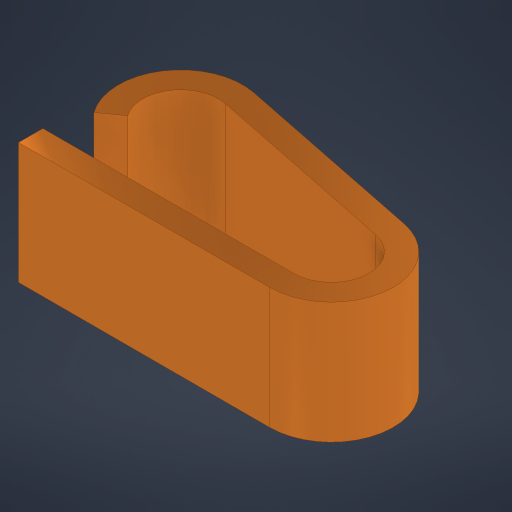
# Autodesk Inventor part: spring contact
Saved by Autodesk Inventor 2024.3 (Build 283343010, 343A)
## iProperties
Created: 2025-05-07
Part Number: spring contact
Material: Gold
Document SubType Name: Modeling
Designer: David
Density: 19.3 g/cm^3
Appearance: Metall - 1600F (heiß)
Author: David
Autodesk Inventor part; units mm, degrees
ref_plane "YZ Plane" through (0, 0, 0) normal (1, 0, 0) x (0, 1, 0)
ref_plane "XZ Plane" through (0, 0, 0) normal (0, 1, 0) x (-1, 0, 0)
ref_plane "XY Plane" through (0, 0, 0) normal (0, 0, 1) x (1, 0, 0)
sketch "Skizze1" plane through (0, 0, 0) normal (0, 0, 1) x (1, 0, 0)
  line L0 (0, 0) -> (2.0711, 0)
  arc A0 (2.0711, 0) -> (2.1726, 1.0089) centre (2.0711, 0.5096) ccw
  line L1 (2.1726, 1.0089) -> (0.6137, 1.3258)
  arc A1 (0.6137, 1.3258) -> (0.0969, 0.5247) centre (0.5117, 0.8243) ccw
  arc A2 (0.5738, 1.1298) -> (0.259, 0.6418) centre (0.5117, 0.8243) ccw
  line L2 (0.5738, 1.1298) -> (2.1327, 0.8129)
  arc A3 (2.0711, 0.2) -> (2.1327, 0.8129) centre (2.0711, 0.5096) ccw
  line L3 (2.0711, 0.2) -> (0, 0.2)
  line L4 (0, 0.2) -> (0, 0)
  line L5 (0.0969, 0.5247) -> (0.259, 0.6418)
  point P0 (0.0806, 1.1)
  point P1 (2.5806, 0.5096)
  dimension "d0" = 0.2
  dimension "d1" = 1.1
  dimension "d2" = 2.5
  constraints: 12 end point, 10 point on circle, 4 centre point, 4 tangent, 1 horizontal, 1 horizontal alignment, 1 line through centre, 1 vertical, 3 other
  measures "d0" distance between parallel lines of L1 L2
  measures "d1" distance from line of L0 point (0.081, 1.1)
  measures "d2" horizontal distance of point (0.081, 1.1) point (2.581, 0.51)
extrude "Extrusion1" add sketch "Skizze1" along normal blind 1
